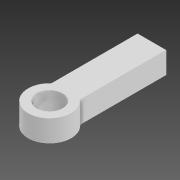
# Autodesk Inventor part: lock
Saved by Autodesk Inventor 2020 (Build 240168000, 168)
## iProperties
Created: 2022-08-26
Part Number: lock
Material: Generic
Document SubType Name: Modeling
Designer: Umair
Density: 1 g/cm^3
Appearance: Default
Author: Umair
Autodesk Inventor part; units mm, degrees
ref_plane "YZ Plane" through (0, 0, 0) normal (1, 0, 0) x (0, 1, 0)
ref_plane "XZ Plane" through (0, 0, 0) normal (0, 1, 0) x (-1, 0, 0)
ref_plane "XY Plane" through (0, 0, 0) normal (0, 0, 1) x (1, 0, 0)
sketch "Sketch1" plane through (0, 0, 0) normal (0, 1, 0) x (-1, 0, 0)
  circle A0 centre (0, 0) radius 3
  circle A1 centre (0, 0) radius 5
  dimension "d0" = 6
  dimension "d1" = 10
  constraints: 2 centre point, 2 coincident
  measures "d0" diameter of A0
  measures "d1" diameter of A1
extrude "Extrusion1" add sketch "Sketch1" along normal blind 5
sketch "Sketch2" plane through (0, 5, 0) normal (0, 1, 0) x (1, 0, 0)
  line L0 (0, 3.7422) -> (-3.316, 3.7422)
  circle A0 centre (0, 0) radius 5 projected
  line L1 (-3.316, 3.7422) -> (-3.316, 23.7422)
  line L2 (-3.316, 3.7422) -> (3.316, 3.7422)
  line L3 (3.316, 3.7422) -> (3.316, 23.7422)
  line L4 (3.316, 23.7422) -> (-3.316, 23.7422)
  dimension "d4" = 20
  constraints: 10 end point, 2 horizontal, 2 perpendicular, 2 point on circle, 1 vertical
  measures "d4" distance of L0.end L1.end
extrude "Extrusion2" add sketch "Sketch2" against normal blind 5 contours L1 L4 L3 A0
body "Solid1"
